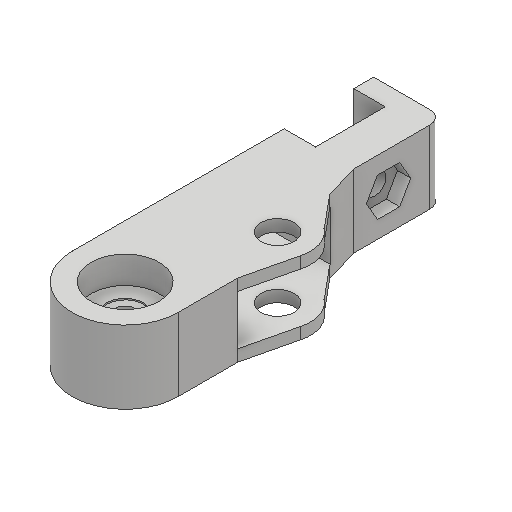
# Autodesk Inventor part: 3DP_ABS_Extruder_Tensioning_Arm
Saved by Autodesk Inventor 2026.1 (Build 301233000, 233)
## iProperties
Created: 2016-01-22
Part Number: 3DP_ABS_Extruder_Tensioning_Arm
Material: Ogólny
Document SubType Name: Modeling
Designer: Andrzej
Density: 1 g/cm^3
Appearance: Default
Mass: 4.47036 g
Surface Area: 37.1093 cm^2
Volume: 4.47036 cm^3
Author: Andrzej
Autodesk Inventor part; units mm, degrees
note: some values were not read from the file. Chosen so that the rebuilt part matches the saved one: edges of "Faza6".
ref_plane "YZ Plane" through (0, 0, 0) normal (1, 0, 0) x (0, 1, 0)
ref_plane "XZ Plane" through (0, 0, 0) normal (0, 1, 0) x (-1, 0, 0)
ref_plane "XY Plane" through (0, 0, 0) normal (0, 0, 1) x (1, 0, 0)
sketch "Szkic1" plane through (0, 0, 0) normal (0, 0, 1) x (1, 0, 0)
  line L0 (-3.8776, -15.6139) -> (12.1224, -15.6139)
  line L1 (12.1224, -15.6139) -> (12.1224, 24.3861)
  line L2 (-3.8776, -15.6139) -> (-3.8776, 24.3861)
  line L3 (-3.8776, 24.3861) -> (12.1224, 24.3861)
  circle A0 centre (4.1224, -7.6139) radius 5.075
  circle A1 centre (4.1224, -7.6139) radius 1.625
  point P0 (0, 0)
  dimension "d0" = 16
  dimension "d1" = 40
  dimension "d2" = 8
  dimension "d3" = 10.15
  dimension "d4" = 8
  dimension "d8" = 3.25
  constraints: 8 end point, 2 centre point, 2 coincident, 2 perpendicular, 1 horizontal, 1 vertical
  measures "d0" distance of L0.start L0.end
  measures "d1" distance of L0.end L1.end
  measures "d2" distance from line of L1 point (4.122, -7.614)
  measures "d3" diameter of A0
  measures "d4" distance from line of L0 A0.centre
  measures "d8" diameter of A1
extrude "Wyciągnięcie proste1" add sketch "Szkic1" along normal blind 11 contours L2 L3 L1 L0 | A0
fillet "Zaokrąglenie1" radius 8 2 edges at (-3.8776, -15.6139, 5.5) (12.1224, -15.6139, 5.5)
sketch "Szkic2" plane through (0, 0, 0) normal (0, 0, -1) x (-1, 0, 0)
  arc A0 (-12.1224, -7.6139) -> (3.8776, -7.6139) centre (-4.1224, -7.6139) ccw projected
  line L0 (-4.1224, -15.6139) -> (-13.9839, -15.6139)
  line L1 (3.8776, 24.3861) -> (3.8776, -7.6139) projected
  circle A1 centre (-9.1224, 10.3861) radius 2.5
  arc A2 (-12.1224, 14.3861) -> (-12.1224, 6.3861) centre (-9.1224, 10.3861) ccw
  arc A3 (-12.1224, -7.6139) -> (3.8776, -7.6139) centre (-4.1224, -7.6139) ccw projected
  line L2 (3.8776, 24.3861) -> (3.8776, -7.6139) projected
  line L3 (-12.1224, 24.3861) -> (3.8776, 24.3861) projected
  line L4 (-12.1224, -7.6139) -> (-12.1224, 24.3861) projected
  line L5 (-12.1224, -7.6139) -> (-12.1224, 24.3861) projected
  line L6 (-12.1224, 19.2527) -> (-8.1224, 19.2527)
  line L7 (-8.1224, 19.2527) -> (-8.1224, 24.3861)
  line L8 (-12.1224, 24.3861) -> (3.8776, 24.3861) projected
  point P0 (0, 0)
  dimension "d10" = 26
  dimension "d13" = 5
  dimension "d14" = 10
  dimension "d16" = 4
  dimension "d23" = 13
  constraints: 6 end point, 4 point on line, 3 point on circle, 2 centre point, 2 perpendicular, 1 coincident, 1 horizontal, 1 tangent
  measures "d10" distance from line of L0 point (-9.122, 10.386)
  measures "d13" diameter of A1
  measures "d14" diameter of A2
  measures "d16" distance of L6.start L6.end
  measures "d23" distance from line of L1 A1.centre
extrude "Wyciągnięcie proste2" add sketch "Szkic2" against normal blind 11 contours A2 L4
extrude "Wyciągnięcie proste3" cut sketch "Szkic2" against normal blind 11.5 contours L4 L3 L7 L6
extrude "Wyciągnięcie proste4" cut sketch "Szkic2" against normal blind 11.5 contours A1
sketch "Szkic3" plane through (-3.8776, 24.3861, 0) normal (-1, 0, 0) x (0, 0, 1)
  line L0 (11, -32) -> (0, -32) projected
  line L1 (11, 0) -> (11, -32) projected
  line L2 (0, 0) -> (11, 0) projected
  line L3 (0, 0) -> (0, -32) projected
  line L4 (1.75, -23) -> (9.25, -23)
  line L5 (1.75, -23) -> (1.75, -5)
  line L6 (1.75, -5) -> (9.25, -5)
  line L7 (9.25, -5) -> (9.25, -23)
  point P0 (0, -24.3861)
  point P1 (5.75, -14)
  dimension "d24" = 14
  dimension "d26" = 9
  dimension "d27" = 7.5
  dimension "d28" = 11
  dimension "d29" = 18
  dimension "d30" = 1.75
  constraints: 8 end point, 1 horizontal, 1 perpendicular, 1 vertical
  measures "d24" distance from line of point (5.75, -14) L2
  measures "d26" distance from line of L4 point (5.75, -14)
  measures "d27" distance of L4.start L4.end
  measures "d28" distance of L2.start L1.start
  measures "d29" distance of L4.start L5.end
  measures "d30" distance between parallel lines of L3 L5
extrude "Wyciągnięcie proste5" cut sketch "Szkic3" against normal blind 20 contours L5 L6 L7 L4
chamfer "Faza3" distance 1.5 distance2 5.1 1 edges at (8.1224, 24.3861, 5.5)
sketch "Szkic5" plane through (0, 0, 0) normal (0, 0, -1) x (-1, 0, 0)
  circle A0 centre (-4.1224, -7.6139) radius 1.625 projected
  circle A1 centre (-4.1224, -7.6139) radius 5.125
  circle A2 centre (-4.1224, -7.6139) radius 2.75
  point P0 (0, 0)
  dimension "d45" = 10.25
  dimension "d64" = 5.5
  constraints: 2 centre point, 2 coincident
  measures "d45" diameter of A1
  measures "d64" diameter of A2
extrude "Wyciągnięcie proste7" cut sketch "Szkic5" against normal blind 4.1 contours A1 | A2
sketch "Szkic6" plane through (0, 0, 11) normal (0, 0, 1) x (1, 0, 0)
  circle A0 centre (4.1224, -7.6139) radius 5.125 projected
  circle A1 centre (4.1224, -7.6139) radius 1.625 projected
  circle A2 centre (4.1224, -7.6139) radius 2.75
  point P0 (0, 0)
  dimension "d67" = 5.5
  constraints: 1 centre point, 1 coincident
  measures "d67" diameter of A2
extrude "Wyciągnięcie proste8" cut sketch "Szkic6" against normal blind 4.1 contours A0 | A2
sketch "Szkic7" plane through (0, 0, 0) normal (0, 0, -1) x (-1, 0, 0)
  circle A0 centre (-4.1224, -7.6139) radius 5.125 projected
  line L0 (-8.1224, 19.2861) -> (-6.6224, 24.3861) projected
  line L1 (-8.1224, 19.2861) -> (-8.1224, 19.2527) projected
  line L2 (-12.1224, 14.3861) -> (-12.1224, 19.2527) projected
  arc A1 (-12.1224, 14.3861) -> (-12.1224, 6.3861) centre (-9.1224, 10.3861) ccw projected
  arc A2 (-12.1224, -7.6139) -> (3.8776, -7.6139) centre (-4.1224, -7.6139) ccw projected
  line L3 (3.8776, 24.3861) -> (3.8776, -7.6139) projected
  line L4 (-6.6224, 24.3861) -> (3.8776, 24.3861) projected
  circle A3 centre (-9.1224, 10.3861) radius 2.5 projected
  line L5 (-6.6224, 24.3861) -> (-6.6224, 37.8861)
  line L6 (-0.8724, 24.3861) -> (-0.8724, 34.8861)
  line L7 (-0.8724, 34.8861) -> (3.8776, 34.8861)
  line L8 (3.8776, 34.8861) -> (3.8776, 37.8861)
  line L9 (3.8776, 37.8861) -> (-6.6224, 37.8861)
  line L10 (-8.1224, 19.2527) -> (-12.1224, 19.2527) projected
  line L11 (-12.1224, -7.6139) -> (-12.1224, 6.3861) projected
  point P0 (0, 0)
  dimension "d50" = 13.5
  dimension "d52" = 5.75
  dimension "d53" = 10.5
  constraints: 10 end point, 2 perpendicular, 2 vertical, 1 horizontal, 1 point on line
  measures "d50" distance of L0.end L5.end
  measures "d52" distance between parallel lines of L6 L5
  measures "d53" distance of L6.start L6.end
extrude "Wyciągnięcie proste9" add sketch "Szkic7" against normal blind 11 contours L5 L9 L8 L7 L6 L4
fillet "Zaokrąglenie2" radius 2 1 edges at (6.6224, 37.8861, 5.5)
chamfer "Faza4" distance 4.8 distance2 4 1 edges at (12.1224, 19.2527, 0.875) measured on face at (12.1224, 16.0083, 0.5833)
chamfer "Faza5" distance 4.8 distance2 4 1 edges at (12.1224, 19.2527, 10.125) measured on face at (12.1224, 16.0083, 9.8333)
extrude "Wyciągnięcie proste10" cut sketch "Szkic5" against normal blind 4.3 contours A2
extrude "Wyciągnięcie proste11" cut sketch "Szkic6" against normal blind 4.3 contours A2
sketch "Szkic9" plane through (0.8724, 24.3861, 0) normal (-1, 0, 0) x (0, 0, 1)
  line L0 (0, 0) -> (0, 10.5) projected
  line L1 (11, 0) -> (0, 0) projected
  line L2 (11, 10.5) -> (11, 0) projected
  line L3 (0, 10.5) -> (11, 10.5) projected
  point P0 (0, -24.3861)
  point P1 (5.5, 5.25)
  dimension "d73" = 5.5
  dimension "d74" = 11
  dimension "d75" = 5.25
  dimension "d76" = 10.5
  measures "d73" distance from line of L0 point (5.5, 5.25)
  measures "d74" distance of L0.end L2.start
  measures "d75" distance from line of L1 point (5.5, 5.25)
  measures "d76" distance between parallel lines of L1 L3
hole "Otwór1" at (0.8724, 29.6361, 5.5) direction (1, 0, 0) diameter 3.25 end through all
sketch "Szkic10" plane through (6.6224, 24.3861, 11) normal (1, 0, 0) x (0, 0, -1)
  circle A0 centre (5.5, 5.25) radius 1.625 projected
  line L0 (0, 11.5) -> (11, 11.5) projected
  line L1 (0, 0) -> (0, 11.5) projected
  line L2 (11, 0) -> (0, 0) projected
  line L3 (11, 11.5) -> (11, 0) projected
  line L4 (8.4, 3.5757) -> (5.5, 1.9014)
  line L5 (5.5, 1.9014) -> (2.6, 3.5757)
  line L6 (2.6, 3.5757) -> (2.6, 6.9243)
  line L7 (2.6, 6.9243) -> (5.5, 8.5986)
  line L8 (5.5, 8.5986) -> (8.4, 6.9243)
  line L9 (8.4, 6.9243) -> (8.4, 3.5757)
  point P0 (11, -24.3861)
  point P1 (8.4, 5.25)
  constraints: 12 end point, 1 midpoint, 13 other
extrude "Wyciągnięcie proste13" cut sketch "Szkic10" against normal blind 2 contours L4 L5 L6 L7 L8 L9
chamfer "Faza6" distance 5 distance2 3.2 1 edges at (12.1224, 6.3861, 0.875)
chamfer "Faza7" [suppressed]
equation "\"d2\" = 0.5 * d0"
equation "\"d26\" = d25"
equation "\"d30\" = -0.5 * d27 + 0.5 * d28"
equation "\"d73\" = 0.5 * d74"
equation "\"d75\" = 0.5 * d76"
equation "\"d25\" = 9"
